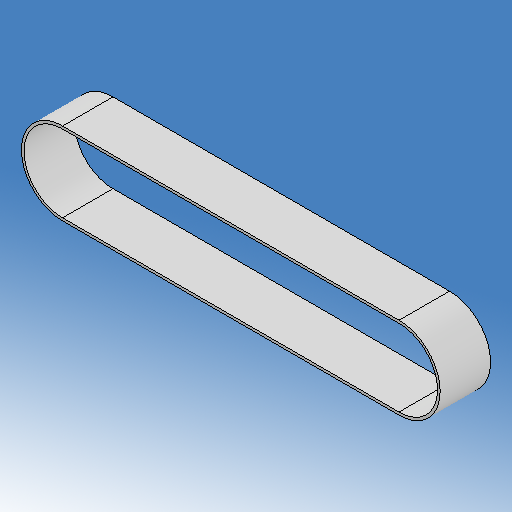
# Autodesk Inventor part: VRT-038Track
Saved by Autodesk Inventor 2025 (Build 290162000, 162)
## iProperties
Created: 2024-06-13
Part Number: VRT-038Track
Material: Generic
Document SubType Name: Modeling
Designer: seene
Density: 1 g/cm^3
Appearance: Default
Author: seene
Autodesk Inventor part; units mm, degrees
ref_plane "YZ Plane" through (0, 0, 0) normal (1, 0, 0) x (0, 1, 0)
ref_plane "XZ Plane" through (0, 0, 0) normal (0, 1, 0) x (-1, 0, 0)
ref_plane "XY Plane" through (0, 0, 0) normal (0, 0, 1) x (1, 0, 0)
sketch "Sketch1" plane through (0, 0, 0) normal (0, 0, 1) x (1, 0, 0)
  line L0 (0, 0) -> (508, 0) construction
  line L1 (0, -58) -> (508, -58)
  line L2 (508, 58) -> (0, 58)
  arc A0 (0, 58) -> (0, -58) centre (0, 0) ccw
  arc A1 (508, -58) -> (508, 58) centre (508, 0) ccw
  line L3 (0, 62) -> (508, 62)
  arc A2 (508, -62) -> (508, 62) centre (508, 0) ccw
  line L4 (508, -62) -> (0, -62)
  arc A3 (0, 62) -> (0, -62) centre (0, 0) ccw
  point P0 (254, 0)
  dimension "d0" = 508
  dimension "d1" = 116
  dimension "d2" = 4
  constraints: 12 end point, 8 point on circle, 4 centre point, 4 tangent, 2 parallel, 1 horizontal, 1 midpoint, 3 other
  measures "d0" distance of L0.start L0.end
  measures "d1" diameter of A1
  measures "d2" distance between parallel lines of L2 L3
extrude "Extrusion1" add sketch "Sketch1" along normal blind 76.2
body "Solid1"
